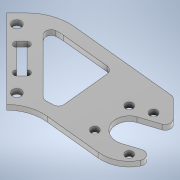
# Autodesk Inventor part: Shoulder_side_frame
Saved by Autodesk Inventor 2020.4 (Build 244396000, 396)
## iProperties
Created: 2022-01-10
Part Number: Shoulder_side_frame
Material: アルミニウム 2014-T4
Document SubType Name: Modeling
Designer: Masato Kubotera
Density: 2.8 g/cm^3
Appearance: 滑らか - 淡い灰色
Description: A2017 T2
Mass: 5.27952 g
Surface Area: 27.5382 cm^2
Volume: 1.88554 cm^3
Author: Masato Kubotera
Autodesk Inventor part; units mm, degrees
ref_plane "YZ Plane" through (0, 0, 0) normal (1, 0, 0) x (0, 1, 0)
ref_plane "XZ Plane" through (0, 0, 0) normal (0, 1, 0) x (-1, 0, 0)
ref_plane "XY Plane" through (0, 0, 0) normal (0, 0, 1) x (1, 0, 0)
sketch "スケッチ1" plane through (0, 0, 0) normal (1, 0, 0) x (0, 1, 0)
  line L0 (-30.3, 41) -> (-30.3, 9)
  line L1 (-30.3, 25) -> (-25.3, 25) construction
  line L2 (-27.8, 31) -> (-25.3, 31) construction
  line L3 (-25.3, 31) -> (-25.3, 19) construction
  line L4 (-25.3, 19) -> (-27.8, 19) construction
  line L5 (-27.8, 19) -> (-27.8, 31) construction
  line L6 (-27.8, 31) -> (-25.3, 19) construction
  line L7 (-25.3, 31) -> (-27.8, 19) construction
  circle A0 centre (-27.8, 37) radius 1.6
  line L8 (-27.8, 70.0011) -> (-27.8, -20.0011) construction
  line L9 (-30.3, 41) -> (-25.3, 41)
  circle A1 centre (0, 0) radius 5.05
  line L10 (0, 8.5) -> (0, -8.5) construction
  circle A2 centre (0, 8.5) radius 1.35
  arc A3 (-7.7075, -7.7075) -> (10.9, 0) centre (0, 0) ccw
  line L11 (-27.85, 31.05) -> (-25.25, 31.05)
  line L12 (-25.25, 31.05) -> (-25.25, 18.95)
  line L13 (-25.25, 18.95) -> (-27.85, 18.95)
  line L14 (-27.85, 18.95) -> (-27.85, 31.05)
  line L15 (-27.85, 31.05) -> (-25.25, 18.95) construction
  line L16 (-25.25, 31.05) -> (-27.85, 18.95) construction
  arc A4 (-25.25, 28.95) -> (-25.25, 31.05) centre (-25.25, 30) ccw
  line L17 (-26.55, 31) -> (-26.55, 19) construction
  arc A5 (-27.85, 31.05) -> (-27.85, 28.95) centre (-27.85, 30) ccw
  arc A6 (-25.25, 18.95) -> (-25.25, 21.05) centre (-25.25, 20) ccw
  arc A7 (-27.85, 21.05) -> (-27.85, 18.95) centre (-27.85, 20) ccw
  circle A8 centre (-27.8, 13) radius 1.6
  line L18 (-13.4742, 36.1016) -> (10.9, 11.7274)
  line L19 (10.9, 11.7274) -> (10.9, 0)
  line L20 (-20.2536, 4.8386) -> (-7.7075, -7.7075)
  circle A9 centre (-6.0104, 6.0104) radius 1.35
  circle A10 centre (-8.5, 0) radius 1.35
  circle A11 centre (0, 0) radius 16 construction
  arc A12 (-13.4742, 36.1016) -> (-25.3, 41) centre (-25.3, 24.2757) ccw
  line L21 (-21.3, 36.3549) -> (-21.3, 10.6202)
  arc A13 (-16.3026, 33.2731) -> (-21.3, 36.3549) centre (-25.3, 24.2757) ccw
  line L22 (6.9, 10.0706) -> (6.9, 8.438)
  circle A14 centre (0, 8.5) radius 2.4 construction
  line L23 (-4.0608, 21.0314) -> (-16.3026, 33.2731)
  arc A15 (-20.2536, 4.8386) -> (-30.3, 9) centre (-30.3, -5.2078) ccw
  circle A16 centre (-6.0104, -6.0104) radius 1.35
  circle A17 centre (0, -8.5) radius 1.35
  arc A18 (-17.4251, 7.6671) -> (-21.3, 10.6202) centre (-30.3, -5.2078) ccw
  line L24 (-17.4251, 7.6671) -> (-4.0608, 21.0314)
  line L25 (-1.9326, -4.6656) -> (6.9917, -8.3622)
  line L26 (1.9326, 4.6656) -> (10.9, 0.9512)
  circle A19 centre (6.0104, -6.0104) radius 1.35
  circle A20 centre (8.5, 0) radius 1.35
  circle A21 centre (6.0104, 6.0104) radius 1.35
  circle A22 centre (-6.0104, 6.0104) radius 2.4 construction
  circle A23 centre (-8.5, 0) radius 2.4 construction
  circle A24 centre (-6.0104, -6.0104) radius 2.4 construction
  circle A25 centre (0, -8.5) radius 2.4 construction
  circle A26 centre (6.0104, -6.0104) radius 2.4 construction
  circle A27 centre (8.5, 0) radius 2.4 construction
  circle A28 centre (6.0104, 6.0104) radius 2.4 construction
  line L27 (6.0104, -6.0104) -> (8.5, 0) construction
  point P0 (-26.55, 25)
  point P1 (-27.8, 25)
  point P2 (0, 5.05)
  point P3 (10.9, 5.05)
  point P4 (0, -5.05)
  point P5 (9.6596, -5.05)
  dimension "d0" = 5
  dimension "d1" = 32
  dimension "d2" = 2.5
  dimension "d3" = 12
  dimension "d4" = 3.2
  dimension "d5" = 5
  dimension "d6" = 10.1
  dimension "d7" = 17
  dimension "d8" = 2.7
  dimension "d10" = 30.3
  dimension "d11" = 1.05
  dimension "d12" = 0.05
  dimension "d13" = 0.05
  dimension "d14" = 24
  dimension "d15" = 25
  dimension "d19" = 360
  dimension "d23" = 32
  dimension "d24" = 45
  dimension "d31" = 4
  dimension "d32" = 4
  dimension "d37" = 4.8
  dimension "d46" = 4
  dimension "d47" = 4
  dimension "d53" = 360
  constraints: 54 end point, 29 centre point, 26 point on circle, 11 midpoint, 9 point on line, 9 tangent, 7 coincident, 7 parallel, 7 symmetric about line, 4 perpendicular, 4 vertical, 3 horizontal, 1 concentric, 1 line through centre, 42 other
  measures "d0" distance of L1.end L1.start
  measures "d1" distance of L0.start L0.end
  measures "d2" distance of L3.end L4.end
  measures "d3" distance of L2.end L3.end
  measures "d4" diameter of A0
  measures "d5" distance of L0.start A12.end
  measures "d6" diameter of A1
  measures "d7" distance of L10.start L10.end
  measures "d8" diameter of A2
  measures "d10" horizontal distance of A1.centre L0.end
  measures "d11" radius of A4
  measures "d12" distance between parallel lines of L2 L11
  measures "d13" distance between parallel lines of L3 L12
  measures "d14" distance of A8.centre A0.centre
  measures "d15" vertical distance of A1.centre L1.start
  measures "d23" diameter of A11
  measures "d24" angle of L0 L18
  measures "d31" distance between parallel lines of L19 L22
  measures "d32" distance between parallel lines of L21 L3
  measures "d37" diameter of A14
  measures "d46" distance between parallel lines of L23 L18
  measures "d47" distance of L20.start L24.start
extrude "押し出し1" add sketch "スケッチ1" along normal blind 2 contours L9 A12 L18 L19 L26 A1 L25 A3 L20 A15 L0 | A9 | A16
fillet "フィレット1" radius 2 4 edges at (1, -21.3, 36.3549) (1, -4.0608, 21.0314) (1, -17.4251, 7.6671) (1, -21.3, 10.6202)
fillet "フィレット2" radius 2 3 edges at (1, 10.9, 11.7274) (1, 6.9917, -8.3622) (1, 10.9, 0.9512)
equation "\"d13\" = d12"
